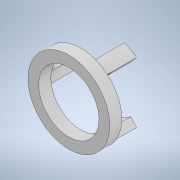
# Autodesk Inventor part: CubeKnob
Saved by Autodesk Inventor 2022 (Build 260153000, 153)
## iProperties
Created: 2022-04-08
Part Number: CubeKnob
Material: Generic
Document SubType Name: Modeling
Designer: awp
Density: 1 g/cm^3
Appearance: Default
Author: awp
Autodesk Inventor part; units mm, degrees
ref_plane "YZ Plane" through (0, 0, 0) normal (1, 0, 0) x (0, 1, 0)
ref_plane "XZ Plane" through (0, 0, 0) normal (0, 1, 0) x (-1, 0, 0)
ref_plane "XY Plane" through (0, 0, 0) normal (0, 0, 1) x (1, 0, 0)
sketch "Sketch1" plane through (0, 0, 0) normal (0, 0, 1) x (1, 0, 0)
  line L0 (28.75, -28.75) -> (-28.75, -28.75) projected
  line L1 (28.75, 28.75) -> (28.75, -28.75) projected
  line L2 (-28.75, 28.75) -> (28.75, 28.75) projected
  line L3 (-28.75, -28.75) -> (-28.75, 28.75) projected
  line L4 (-21.13, -17.2033) -> (-17.2033, -17.2033) projected
  line L5 (-17.2033, -17.2033) -> (-17.2033, -21.13) projected
  line L6 (-17.2033, -21.13) -> (-21.13, -21.13) projected
  line L7 (-21.13, -21.13) -> (-21.13, -17.2033) projected
  line L8 (-1.9633, 17.2033) -> (-1.9633, 21.13) projected
  line L9 (-1.9633, 21.13) -> (1.9633, 21.13) projected
  line L10 (1.9633, 21.13) -> (1.9633, 17.2033) projected
  line L11 (1.9633, 17.2033) -> (0, 17.2033) projected
  arc A0 (16.754, 3.9061) -> (0, 17.2033) centre (0, 0) ccw projected
  arc A1 (16.0426, 2.8287) -> (16.754, 3.9061) centre (15.8882, 3.7042) ccw projected
  line L12 (16.0426, 2.8287) -> (13.3539, 2.3547) projected
  arc A2 (12.336, 3.0188) -> (13.3539, 2.3547) centre (13.1995, 3.2301) ccw projected
  arc A3 (12.336, 3.0188) -> (-3.5536, 12.1927) centre (0, 0) ccw projected
  arc A4 (-4.6378, 12.7421) -> (-3.5536, 12.1927) centre (-3.8024, 13.0462) ccw projected
  line L13 (-4.6378, 12.7421) -> (-5.5715, 15.3077) projected
  arc A5 (-4.9942, 16.4625) -> (-5.5715, 15.3077) centre (-4.7362, 15.6117) ccw projected
  arc A6 (0, 17.2033) -> (-4.9942, 16.4625) centre (0, 0) ccw projected
  line L14 (0, 17.2033) -> (-1.9633, 17.2033) projected
  line L15 (17.2033, -21.13) -> (17.2033, -17.2033) projected
  line L16 (17.2033, -17.2033) -> (21.13, -17.2033) projected
  line L17 (21.13, -17.2033) -> (21.13, -21.13) projected
  line L18 (21.13, -21.13) -> (17.2033, -21.13) projected
  line L19 (-21.13, 17.2033) -> (-21.13, 21.13) projected
  line L20 (-21.13, 21.13) -> (-17.2033, 21.13) projected
  line L21 (-17.2033, 21.13) -> (-17.2033, 17.2033) projected
  line L22 (-17.2033, 17.2033) -> (-21.13, 17.2033) projected
  line L23 (-21.13, -1.9633) -> (-21.13, 1.9633) projected
  line L24 (-21.13, 1.9633) -> (-17.2033, 1.9633) projected
  line L25 (-17.2033, 1.9633) -> (-17.2033, 0) projected
  arc A7 (-11.7598, 12.5564) -> (-17.2033, 0) centre (0, 0) ccw projected
  arc A8 (-10.4711, 12.4789) -> (-11.7598, 12.5564) centre (-11.1521, 11.9075) ccw projected
  line L26 (-10.4711, 12.4789) -> (-8.7161, 10.3875) projected
  arc A9 (-8.7824, 9.1739) -> (-8.7161, 10.3875) centre (-9.3971, 9.816) ccw projected
  arc A10 (-8.7824, 9.1739) -> (-8.7824, -9.1739) centre (0, 0) ccw projected
  arc A11 (-8.7161, -10.3875) -> (-8.7824, -9.1739) centre (-9.3971, -9.816) ccw projected
  line L27 (-8.7161, -10.3875) -> (-10.4711, -12.4789) projected
  arc A12 (-11.7598, -12.5564) -> (-10.4711, -12.4789) centre (-11.1521, -11.9075) ccw projected
  arc A13 (-17.2033, 0) -> (-11.7598, -12.5564) centre (0, 0) ccw projected
  line L28 (-17.2033, 0) -> (-17.2033, -1.9633) projected
  line L29 (-17.2033, -1.9633) -> (-21.13, -1.9633) projected
  line L30 (-1.9633, -1.9633) -> (-1.9633, 1.9633) projected
  line L31 (-1.9633, 1.9633) -> (1.9633, 1.9633) projected
  line L32 (1.9633, 1.9633) -> (1.9633, -1.9633) projected
  line L33 (1.9633, -1.9633) -> (-1.9633, -1.9633) projected
  line L34 (17.2033, -1.9633) -> (17.2033, 1.9633) projected
  line L35 (17.2033, 1.9633) -> (21.13, 1.9633) projected
  line L36 (21.13, 1.9633) -> (21.13, -1.9633) projected
  line L37 (21.13, -1.9633) -> (17.2033, -1.9633) projected
  line L38 (17.2033, 17.2033) -> (17.2033, 21.13) projected
  line L39 (17.2033, 21.13) -> (21.13, 21.13) projected
  line L40 (21.13, 21.13) -> (21.13, 17.2033) projected
  line L41 (21.13, 17.2033) -> (17.2033, 17.2033) projected
  line L42 (-1.9633, -21.13) -> (-1.9633, -17.2033) projected
  line L43 (-1.9633, -17.2033) -> (0, -17.2033) projected
  arc A14 (-4.9942, -16.4625) -> (0, -17.2033) centre (0, 0) ccw projected
  arc A15 (-5.5715, -15.3077) -> (-4.9942, -16.4625) centre (-4.7362, -15.6117) ccw projected
  line L44 (-5.5715, -15.3077) -> (-4.6378, -12.7421) projected
  arc A16 (-3.5536, -12.1927) -> (-4.6378, -12.7421) centre (-3.8024, -13.0462) ccw projected
  arc A17 (-3.5536, -12.1927) -> (12.336, -3.0188) centre (0, 0) ccw projected
  arc A18 (13.3539, -2.3547) -> (12.336, -3.0188) centre (13.1995, -3.2301) ccw projected
  line L45 (13.3539, -2.3547) -> (16.0426, -2.8287) projected
  arc A19 (16.754, -3.9061) -> (16.0426, -2.8287) centre (15.8882, -3.7042) ccw projected
  arc A20 (0, -17.2033) -> (16.754, -3.9061) centre (0, 0) ccw projected
  line L46 (0, -17.2033) -> (1.9633, -17.2033) projected
  line L47 (1.9633, -17.2033) -> (1.9633, -21.13) projected
  line L48 (1.9633, -21.13) -> (-1.9633, -21.13) projected
  circle A21 centre (0, 0) radius 17.2033
  circle A22 centre (0, 0) radius 12.7
  line L49 (0, 0) -> (-16.942, 2.9873)
  line L50 (0, 0) -> (17.2033, 0) construction
  line L51 (0, 0) -> (-16.942, -2.9873)
  line L52 (0, 0) -> (17.2033, 0) construction
  line L53 (0, 0) -> (11.0581, -13.1785)
  line L54 (0, 0) -> (17.2033, 0) construction
  line L55 (0, 0) -> (5.6822, -15.6117)
  line L56 (0, 0) -> (16.6137, 0) construction
  line L57 (5.6822, -15.6117) -> (5.8839, -16.1658)
  line L58 (0, 0) -> (11.0581, 13.1785)
  line L59 (0, 0) -> (17.2033, 0) construction
  line L60 (0, 0) -> (5.8839, 16.1658)
  line L61 (0, 0) -> (17.2033, 0) construction
  point P0 (-4.9942, -16.4625)
  point P1 (16.754, 3.9061)
  point P2 (12.336, -3.0188)
  point P3 (-8.7824, -9.1739)
  point P4 (-3.5536, 12.1927)
  dimension "d0" = 170
  dimension "d1" = 170
  dimension "d2" = 50
  dimension "d3" = 70
  dimension "d4" = 50
  dimension "d5" = 70
  constraints: 26 end point, 6 equal length, 6 horizontal, 6 point on circle, 2 centre point, 2 coincident, 2 concentric, 1 point on line
  measures "d0" angle of L50 L49
  measures "d1" angle of L51 L52
  measures "d2" angle of L53 L54
  measures "d3" angle of L55 L56
  measures "d4" angle of L59 L58
  measures "d5" angle of L61 L60
extrude "Extrusion1" add sketch "Sketch1" along normal blind 5.08 contours A0 L60 A3 A4 L13 A5 A6 | A0 L58 A3 L60 | A5 L13 A4 A22 A9 L26 A8 A21 | A0 A1 L12 A2 A3 L58 | A8 L26 A9 A10 L49 A7 | A21 A19 L45 A18 A22 A2 L12 A1 | L49 A10 L51 A13 A7 | A20 L53 A17 A18 L45 A19 | L51 A10 A11 L27 A12 A13 | A20 L57 L55 A17 L53 | L55 L57 A20 A14 A15 L44 A16 A17 | A12 L27 A11 A22 A16 L44 A15 A21
ref_plane "Work Plane1" through (0, 0, 0) normal (0, 0, 1) x (1, 0, 0)
sketch "Sketch3" plane through (0, 0, 0) normal (0, 0, 1) x (1, 0, 0)
  line L0 (28.75, -28.75) -> (-28.75, -28.75)
  line L1 (28.75, 28.75) -> (28.75, -28.75)
  line L2 (-28.75, 28.75) -> (28.75, 28.75)
  line L3 (-28.75, -28.75) -> (-28.75, 28.75)
  line L4 (-21.13, -17.2033) -> (-17.2033, -17.2033)
  line L5 (-17.2033, -17.2033) -> (-17.2033, -21.13)
  line L6 (-17.2033, -21.13) -> (-21.13, -21.13)
  line L7 (-21.13, -21.13) -> (-21.13, -17.2033)
  line L8 (-1.9633, 17.2033) -> (-1.9633, 21.13)
  line L9 (-1.9633, 21.13) -> (1.9633, 21.13)
  line L10 (1.9633, 21.13) -> (1.9633, 17.2033)
  line L11 (1.9633, 17.2033) -> (0, 17.2033)
  arc A0 (16.754, 3.9061) -> (0, 17.2033) centre (0, 0) ccw
  arc A1 (16.0426, 2.8287) -> (16.754, 3.9061) centre (15.8882, 3.7042) ccw
  line L12 (16.0426, 2.8287) -> (13.3539, 2.3547)
  arc A2 (12.336, 3.0188) -> (13.3539, 2.3547) centre (13.1995, 3.2301) ccw
  arc A3 (12.336, 3.0188) -> (-3.5536, 12.1927) centre (0, 0) ccw
  arc A4 (-4.6378, 12.7421) -> (-3.5536, 12.1927) centre (-3.8024, 13.0462) ccw
  line L13 (-4.6378, 12.7421) -> (-5.5715, 15.3077)
  arc A5 (-4.9942, 16.4625) -> (-5.5715, 15.3077) centre (-4.7362, 15.6117) ccw
  arc A6 (0, 17.2033) -> (-4.9942, 16.4625) centre (0, 0) ccw
  line L14 (0, 17.2033) -> (-1.9633, 17.2033)
  line L15 (17.2033, -21.13) -> (17.2033, -17.2033)
  line L16 (17.2033, -17.2033) -> (21.13, -17.2033)
  line L17 (21.13, -17.2033) -> (21.13, -21.13)
  line L18 (21.13, -21.13) -> (17.2033, -21.13)
  line L19 (-21.13, 17.2033) -> (-21.13, 21.13)
  line L20 (-21.13, 21.13) -> (-17.2033, 21.13)
  line L21 (-17.2033, 21.13) -> (-17.2033, 17.2033)
  line L22 (-17.2033, 17.2033) -> (-21.13, 17.2033)
  line L23 (-21.13, -1.9633) -> (-21.13, 1.9633)
  line L24 (-21.13, 1.9633) -> (-17.2033, 1.9633)
  line L25 (-17.2033, 1.9633) -> (-17.2033, 0)
  arc A7 (-11.7598, 12.5564) -> (-17.2033, 0) centre (0, 0) ccw
  arc A8 (-10.4711, 12.4789) -> (-11.7598, 12.5564) centre (-11.1521, 11.9075) ccw
  line L26 (-10.4711, 12.4789) -> (-8.7161, 10.3875)
  arc A9 (-8.7824, 9.1739) -> (-8.7161, 10.3875) centre (-9.3971, 9.816) ccw
  arc A10 (-8.7824, 9.1739) -> (-8.7824, -9.1739) centre (0, 0) ccw
  arc A11 (-8.7161, -10.3875) -> (-8.7824, -9.1739) centre (-9.3971, -9.816) ccw
  line L27 (-8.7161, -10.3875) -> (-10.4711, -12.4789)
  arc A12 (-11.7598, -12.5564) -> (-10.4711, -12.4789) centre (-11.1521, -11.9075) ccw
  arc A13 (-17.2033, 0) -> (-11.7598, -12.5564) centre (0, 0) ccw
  line L28 (-17.2033, 0) -> (-17.2033, -1.9633)
  line L29 (-17.2033, -1.9633) -> (-21.13, -1.9633)
  line L30 (-1.9633, -1.9633) -> (-1.9633, 1.9633)
  line L31 (-1.9633, 1.9633) -> (1.9633, 1.9633)
  line L32 (1.9633, 1.9633) -> (1.9633, -1.9633)
  line L33 (1.9633, -1.9633) -> (-1.9633, -1.9633)
  line L34 (17.2033, -1.9633) -> (17.2033, 1.9633)
  line L35 (17.2033, 1.9633) -> (21.13, 1.9633)
  line L36 (21.13, 1.9633) -> (21.13, -1.9633)
  line L37 (21.13, -1.9633) -> (17.2033, -1.9633)
  line L38 (17.2033, 17.2033) -> (17.2033, 21.13)
  line L39 (17.2033, 21.13) -> (21.13, 21.13)
  line L40 (21.13, 21.13) -> (21.13, 17.2033)
  line L41 (21.13, 17.2033) -> (17.2033, 17.2033)
  line L42 (-1.9633, -21.13) -> (-1.9633, -17.2033)
  line L43 (-1.9633, -17.2033) -> (0, -17.2033)
  arc A14 (-4.9942, -16.4625) -> (0, -17.2033) centre (0, 0) ccw
  arc A15 (-5.5715, -15.3077) -> (-4.9942, -16.4625) centre (-4.7362, -15.6117) ccw
  line L44 (-5.5715, -15.3077) -> (-4.6378, -12.7421)
  arc A16 (-3.5536, -12.1927) -> (-4.6378, -12.7421) centre (-3.8024, -13.0462) ccw
  arc A17 (-3.5536, -12.1927) -> (12.336, -3.0188) centre (0, 0) ccw
  arc A18 (13.3539, -2.3547) -> (12.336, -3.0188) centre (13.1995, -3.2301) ccw
  line L45 (13.3539, -2.3547) -> (16.0426, -2.8287)
  arc A19 (16.754, -3.9061) -> (16.0426, -2.8287) centre (15.8882, -3.7042) ccw
  arc A20 (0, -17.2033) -> (16.754, -3.9061) centre (0, 0) ccw
  line L46 (0, -17.2033) -> (1.9633, -17.2033)
  line L47 (1.9633, -17.2033) -> (1.9633, -21.13)
  line L48 (1.9633, -21.13) -> (-1.9633, -21.13)
  circle A21 centre (0, 0) radius 17.2033
  circle A22 centre (0, 0) radius 12.7
  line L49 (0, 0) -> (-16.942, 2.9873)
  line L50 (0, 0) -> (17.2033, 0) construction
  line L51 (0, 0) -> (-16.942, -2.9873)
  line L52 (0, 0) -> (17.2033, 0) construction
  line L53 (0, 0) -> (11.0581, -13.1785)
  line L54 (0, 0) -> (17.2033, 0) construction
  line L55 (0, 0) -> (5.6822, -15.6117)
  line L56 (0, 0) -> (16.6137, 0) construction
  line L57 (5.6822, -15.6117) -> (5.8839, -16.1658)
  line L58 (0, 0) -> (11.0581, 13.1785)
  line L59 (0, 0) -> (17.2033, 0) construction
  line L60 (0, 0) -> (5.8839, 16.1658)
  line L61 (0, 0) -> (17.2033, 0) construction
  circle A23 centre (0, 0) radius 16.7005
  circle A24 centre (0, 0) radius 13.0175
  point P0 (-4.9942, -16.4625)
  point P1 (16.754, 3.9061)
  point P2 (12.336, -3.0188)
  point P3 (-8.7824, -9.1739)
  point P4 (-3.5536, 12.1927)
  point P5 (8.1634, -9.7288)
  point P6 (4.3437, -11.9341)
  point P7 (-12.5071, -2.2053)
  point P8 (-12.5071, 2.2053)
  point P9 (4.3437, 11.9341)
  point P10 (8.1634, 9.7288)
  point P11 (4.4522, 12.2324)
  point P12 (8.3675, 9.972)
  point P13 (10.7349, 12.7933)
  point P14 (5.7119, 15.6933)
  point P15 (-12.8197, -2.2605)
  point P16 (-12.8197, 2.2605)
  point P17 (-16.4468, 2.9)
  point P18 (-16.4468, -2.9)
  point P19 (8.3675, -9.972)
  point P20 (4.4522, -12.2324)
  point P21 (5.7119, -15.6933)
  point P22 (10.7349, -12.7933)
  dimension "d8" = 170
  dimension "d9" = 170
  dimension "d10" = 50
  dimension "d11" = 70
  dimension "d12" = 50
  dimension "d13" = 70
  dimension "d16" = 33.401
  dimension "d17" = 26.035
  constraints: 124 end point, 48 point on circle, 25 centre point, 6 equal length, 6 horizontal, 4 coincident, 2 concentric, 1 point on line
  measures "d8" angle of L50 L49
  measures "d9" angle of L51 L52
  measures "d10" angle of L53 L54
  measures "d11" angle of L55 L56
  measures "d12" angle of L59 L58
  measures "d13" angle of L61 L60
  measures "d16" diameter of A23
  measures "d17" diameter of A24
extrude "Extrusion2" add sketch "Sketch3" against normal blind 12.7 contours A23 L58 A24 L60 | L49 A24 L51 A23 | A23 L57 L55 A24 L53
sketch "Sketch4" plane through (0, 0, -12.7) normal (0, 0, -1) x (-1, 0, 0)
  line L0 (-10.7349, 12.7933) -> (-8.3675, 9.972) projected
  arc A0 (-4.4522, 12.2324) -> (-8.3675, 9.972) centre (0, 0) ccw projected
  line L1 (-4.4522, 12.2324) -> (-5.7119, 15.6933) projected
  arc A1 (-5.7119, 15.6933) -> (-10.7349, 12.7933) centre (0, 0) ccw projected
  line L2 (16.4468, 2.9) -> (12.8197, 2.2605) projected
  arc A2 (12.8197, -2.2605) -> (12.8197, 2.2605) centre (0, 0) ccw projected
  line L3 (12.8197, -2.2605) -> (16.4468, -2.9) projected
  arc A3 (16.4468, -2.9) -> (16.4468, 2.9) centre (0, 0) ccw projected
  line L4 (-5.7119, -15.6933) -> (-4.4522, -12.2324) projected
  arc A4 (-8.3675, -9.972) -> (-4.4522, -12.2324) centre (0, 0) ccw projected
  line L5 (-8.3675, -9.972) -> (-10.7349, -12.7933) projected
  arc A5 (-10.7349, -12.7933) -> (-5.7119, -15.6933) centre (0, 0) ccw projected
  circle A6 centre (0, 0) radius 14.9225
  circle A7 centre (-7.5175, 12.8906) radius 1.5
  circle A8 centre (14.9225, 0) radius 1.5
  circle A9 centre (-7.5175, -12.8906) radius 1.5
  dimension "d18" = 3
  dimension "d19" = 3
  dimension "d20" = 3
  constraints: 4 centre point, 3 point on circle, 1 coincident
  measures "d18" diameter of A7
  measures "d19" diameter of A8
  measures "d20" diameter of A9
extrude "Extrusion3" cut sketch "Sketch4" against normal blind 6.35 contours A7 A6 | A6 A7 | A9 A6 | A6 A9 | A8 A6 | A6 A8
body "Solid1"
